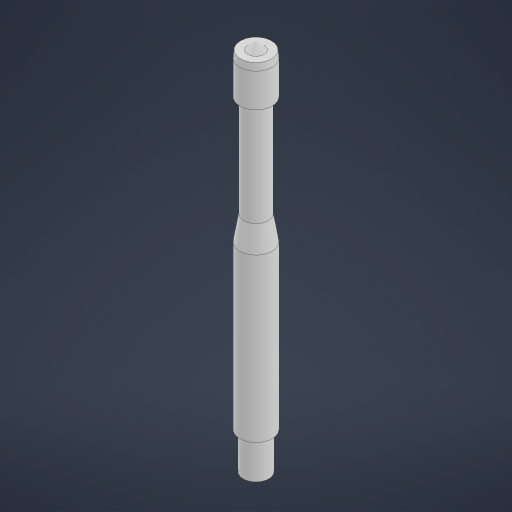
# Autodesk Inventor part: DORMER_SPU4908_M8SpiralFl_TAP
Saved by Autodesk Inventor 2024.3 (Build 283343000, 343)
## iProperties
Created: 2024-06-20
Part Number: DORMER_SPU4908_M8SpiralFl_TAP
Material: Generic
Document SubType Name: Modeling
Designer: fablabadmin
Density: 1 g/cm^3
Appearance: Default
Author: fablabadmin
Autodesk Inventor part; units mm, degrees
ref_plane "YZ Plane" through (0, 0, 0) normal (1, 0, 0) x (0, 1, 0)
ref_plane "XZ Plane" through (0, 0, 0) normal (0, 1, 0) x (-1, 0, 0)
ref_plane "XY Plane" through (0, 0, 0) normal (0, 0, 1) x (1, 0, 0)
sketch "Sketch1" plane through (0, 0, 0) normal (0, 0, 1) x (1, 0, 0)
  line L0 (-4.8, 0) -> (0.8, 0) construction
  line L1 (0, -18.4) -> (0, 110.4) projected
  line L2 (-3.15, 0) -> (-3.15, 9)
  line L3 (-3.15, 9) -> (-4, 9)
  line L4 (-4, 9) -> (-4, 49)
  line L5 (-4, 49) -> (-3, 55)
  line L6 (-3, 55) -> (-3, 80)
  line L7 (-3, 80) -> (-4, 80)
  line L8 (-4, 80) -> (-4, 88.25)
  line L9 (-4, 88.25) -> (-3.8469, 90)
  line L10 (-3.8469, 90) -> (-2, 90)
  line L11 (-2, 90) -> (0, 92)
  line L12 (0, 92) -> (0, 0)
  line L13 (-3.15, 0) -> (0, 0)
  dimension "d1" = 92
  dimension "d2" = 8
  dimension "d4" = 6
  dimension "d16" = 45
  dimension "d18" = 3.75
  dimension "d19" = 12
  dimension "d20" = 37
  dimension "d21" = 43
  dimension "d22" = 5
  dimension "d23" = 2
  dimension "d24" = 8
  dimension "d28" = 6.3
  dimension "d29" = 9
  constraints: 24 end point, 3 perpendicular, 2 collinear, 2 point on line, 2 vertical, 1 horizontal, 1 parallel
  measures "d1" distance of L12.end L11.end
  measures "d2" diameter of L4 L1
  measures "d4" diameter of L6 L1
  measures "d16" angle of L10 L11
  measures "d18" vertical distance of L8.end L11.end
  measures "d19" vertical distance of L7.end L11.end
  measures "d20" vertical distance of L5.end L11.end
  measures "d21" vertical distance of L4.end L11.end
  measures "d22" angle of L8 L9
  measures "d23" distance from line of L11.end L10
  measures "d24" diameter of L8 L1
  measures "d28" diameter of L2 L1
  measures "d29" distance of L2.start L2.end
revolve "Revolution2" add sketch "Sketch1" angle 360 about axis through (0, -10, 0) along (0, 1, 0)
body "Solid2"
